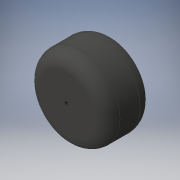
# Autodesk Inventor part: flyWheel
Saved by Autodesk Inventor 2016 (Build 200138000, 138)
## iProperties
Created: 2015-11-01
Part Number: flyWheel
Material: Generic
Document SubType Name: Modeling
Designer: rossmosier
Density: 1 g/cm^3
Appearance: Rubber - Black
Author: rossmosier
Autodesk Inventor part; units mm, degrees
ref_plane "YZ Plane" through (0, 0, 0) normal (1, 0, 0) x (0, 1, 0)
ref_plane "XZ Plane" through (0, 0, 0) normal (0, 1, 0) x (-1, 0, 0)
ref_plane "XY Plane" through (0, 0, 0) normal (0, 0, 1) x (1, 0, 0)
sketch "Sketch2" plane through (0, 0, 0) normal (0, 0, 1) x (1, 0, 0)
  circle A0 centre (0, 0) radius 76.2
  circle A1 centre (0, 0) radius 3.175
  dimension "d0" = 152.4
  dimension "d1" = 6.35
  constraints: 2 centre point, 2 coincident
  measures "d0" diameter of A0
  measures "d1" diameter of A1
extrude "Extrusion1" add sketch "Sketch2" along normal blind 88.9
fillet "Fillet1" radius 25.4 2 edges at (-76.2, 0, 88.9) (-76.2, 0, 0)
body "Solid1"
